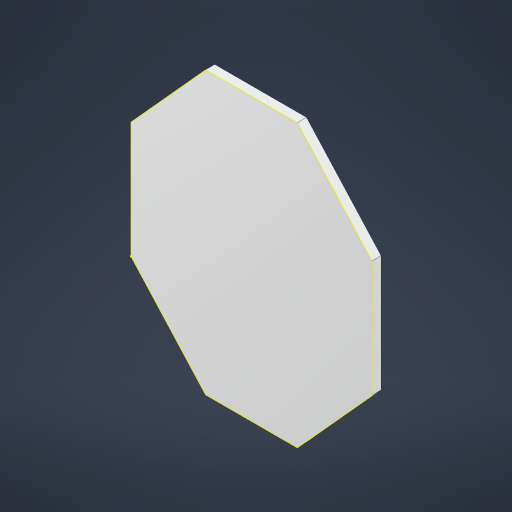
# Autodesk Inventor part: DVBS_008_bellypan
Saved by Autodesk Inventor 2024 (Build 280153000, 153)
## iProperties
Created: 2024-07-31
Part Number: DVBS_008_bellypan
Material: Aluminum 6061
Document SubType Name: Modeling
Designer: sarav
Density: 2.7 g/cm^3
Appearance: Aluminum - Flat
Author: sarav
Autodesk Inventor part; units mm, degrees
ref_plane "YZ Plane" through (0, 0, 0) normal (1, 0, 0) x (0, 1, 0)
ref_plane "XZ Plane" through (0, 0, 0) normal (0, 1, 0) x (-1, 0, 0)
ref_plane "XY Plane" through (0, 0, 0) normal (0, 0, 1) x (1, 0, 0)
sketch "Sketch1" plane through (0, 0, 0) normal (0, 0, 1) x (1, 0, 0)
  line L0 (0, 0) -> (0, 317.5)
  line L1 (0, 317.5) -> (203.2, 317.5) construction
  line L2 (203.2, 317.5) -> (203.2, 542.3916) construction
  line L3 (0, 317.5) -> (203.2, 542.3916)
  line L4 (203.2, 542.3916) -> (453.4916, 542.3916)
  line L5 (453.4916, 542.3916) -> (453.4916, 317.5) construction
  line L6 (453.4916, 317.5) -> (656.6916, 317.5) construction
  line L7 (656.6916, 317.5) -> (453.4916, 542.3916)
  line L8 (0, 0) -> (203.2, 0) construction
  line L9 (203.2, 0) -> (203.2, -224.8916) construction
  line L10 (203.2, -224.8916) -> (0, 0)
  line L11 (203.2, -224.8916) -> (453.4916, -224.8916)
  line L12 (453.4916, -224.8916) -> (453.4916, 0) construction
  line L13 (453.4916, 0) -> (656.6916, 0) construction
  line L14 (656.6916, 0) -> (453.4916, -224.8916)
  line L15 (656.6916, 317.5) -> (656.6916, 0)
  dimension "d0" = 317.5
  dimension "d1" = 203.2
  dimension "d2" = 224.8916
  dimension "d3" = 250.2916
  dimension "d4" = 224.8916
  dimension "d5" = 203.2
  dimension "d6" = 203.2
  dimension "d7" = 224.8916
  dimension "d8" = 250.2916
  dimension "d9" = 203.2
  constraints: 32 end point, 4 perpendicular, 4 vertical, 3 horizontal, 1 parallel
  measures "d0" distance of L0.start L0.end
  measures "d1" distance of L0.end L1.end
  measures "d2" distance of L1.end L2.end
  measures "d3" distance of L2.end L4.end
  measures "d4" distance of L4.end L5.end
  measures "d5" distance of L5.end L6.end
  measures "d6" distance of L0.start L8.end
  measures "d7" distance of L8.end L9.end
  measures "d8" distance of L9.end L11.end
  measures "d9" distance of L12.end L13.end
extrude "Extrusion1" add sketch "Sketch1" along normal blind 25.4
sketch "Sketch2" plane through (0, 0, 25.4) normal (0, 0, 1) x (1, 0, 0)
  line L0 (453.4916, -224.8916) -> (656.6916, 0) projected
  line L1 (656.6916, 0) -> (656.6916, 317.5) projected
  line L2 (656.6916, 317.5) -> (453.4916, 542.3916) projected
  line L3 (453.4916, 542.3916) -> (203.2, 542.3916) projected
  line L4 (203.2, 542.3916) -> (0, 317.5) projected
  line L5 (0, 317.5) -> (0, 0) projected
  line L6 (0, 0) -> (203.2, -224.8916) projected
  line L7 (203.2, -224.8916) -> (453.4916, -224.8916) projected
  line L8 (453.4916, 542.3916) -> (203.2, 542.3916) projected
body "Solid1"
